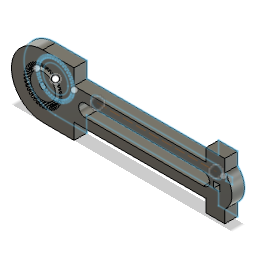
top slider mod v1 (Autodesk Fusion 360 design; units mm, degrees)
Autodesk Fusion 360 part; units mm, degrees
sketch "Sketch1" plane through (0, 0, 0) normal (0, 0, 1) x (1, 0, 0)
  line L0 (100.0107, 100.3168) -> (205.0107, 100.3168)
  line L1 (205.0107, 75.3168) -> (100.0107, 75.3168)
  line L2 (100.0107, 100.3168) -> (100.0107, 112.8168)
  line L3 (100.0107, 112.8168) -> (75.2033, 112.8168)
  line L4 (75.1963, 62.8169) -> (100.0107, 62.8169)
  line L5 (100.0107, 62.8169) -> (100.0107, 75.3168)
  arc A0 (75.2033, 112.8168) -> (75.1963, 62.8169) centre (75.2032, 87.8168) ccw
  circle A1 centre (75.2032, 87.8168) radius 10
  line L6 (74.5404, 102.8022) -> (74.8532, 100.8268)
  line L7 (74.8532, 100.8268) -> (75.5532, 100.8268)
  line L8 (75.5532, 100.8268) -> (75.9001, 102.8007)
  line L9 (72.1452, 102.5018) -> (72.7708, 100.6022)
  line L10 (72.7708, 100.6022) -> (73.4618, 100.7145)
  line L11 (73.4618, 100.7145) -> (73.4875, 102.7184)
  line L12 (69.8292, 101.8211) -> (70.7514, 100.0464)
  line L13 (70.7514, 100.0464) -> (71.4154, 100.2681)
  line L14 (71.4154, 100.2681) -> (71.1193, 102.2502)
  line L15 (67.6523, 100.7777) -> (68.8473, 99.1739)
  line L16 (68.8473, 99.1739) -> (69.4671, 99.4993)
  line L17 (69.4671, 99.4993) -> (68.8569, 101.4082)
  line L18 (65.671, 99.3986) -> (67.1078, 98.0073)
  line L19 (67.1078, 98.0073) -> (67.6674, 98.4278)
  line L20 (67.6674, 98.4278) -> (66.7589, 100.2142)
  line L21 (63.9366, 97.7196) -> (65.578, 96.5767)
  line L22 (65.578, 96.5767) -> (66.0629, 97.0816)
  line L23 (66.0629, 97.0816) -> (64.8796, 98.6991)
  line L24 (62.494, 95.784) -> (64.2974, 94.9193)
  line L25 (64.2974, 94.9193) -> (64.6951, 95.4954)
  line L26 (64.6951, 95.4954) -> (63.2677, 96.9021)
  line L27 (61.3806, 93.6422) -> (63.2993, 93.0779)
  line L28 (63.2993, 93.0779) -> (63.5994, 93.7103)
  line L29 (63.5994, 93.7103) -> (61.9648, 94.8699)
  line L30 (60.6251, 91.3494) -> (62.6095, 91.1003)
  line L31 (62.6095, 91.1003) -> (62.8043, 91.7726)
  line L32 (62.8043, 91.7726) -> (61.0049, 92.6549)
  line L33 (60.2472, 88.9652) -> (62.2459, 89.0376)
  line L34 (62.2459, 89.0376) -> (62.3303, 89.7325)
  line L35 (62.3303, 89.7325) -> (60.4127, 90.3147)
  line L36 (60.2567, 86.5512) -> (62.2179, 86.9433)
  line L37 (62.2179, 86.9433) -> (62.1897, 87.6427)
  line L38 (62.1897, 87.6427) -> (60.2035, 87.9098)
  line L39 (60.6533, 84.17) -> (62.5262, 84.8716)
  line L40 (62.5262, 84.8716) -> (62.3862, 85.5574)
  line L41 (62.3862, 85.5574) -> (60.3828, 85.5025)
  line L42 (61.4267, 81.8832) -> (63.1628, 82.8762)
  line L43 (63.1628, 82.8762) -> (62.9146, 83.5307)
  line L44 (62.9146, 83.5307) -> (60.946, 83.1551)
  line L45 (62.5569, 79.7502) -> (64.1113, 81.0088)
  line L46 (64.1113, 81.0088) -> (63.7613, 81.615)
  line L47 (63.7613, 81.615) -> (61.8784, 80.9284)
  line L48 (64.0147, 77.826) -> (65.347, 79.3176)
  line L49 (65.347, 79.3176) -> (64.9043, 79.8599)
  line L50 (64.9043, 79.8599) -> (63.156, 78.8802)
  line L51 (65.7622, 76.1606) -> (66.838, 77.8467)
  line L52 (66.838, 77.8467) -> (66.3141, 78.3108)
  line L53 (66.3141, 78.3108) -> (64.7455, 77.0634)
  line L54 (67.7543, 74.7971) -> (68.5457, 76.6339)
  line L55 (68.5457, 76.6339) -> (67.954, 77.008)
  line L56 (67.954, 77.008) -> (66.6059, 75.5251)
  line L57 (69.9392, 73.7708) -> (70.4258, 75.7108)
  line L58 (70.4258, 75.7108) -> (69.7818, 75.9851)
  line L59 (69.7818, 75.9851) -> (68.689, 74.3052)
  line L60 (72.2605, 73.1083) -> (72.4296, 75.1012)
  line L61 (72.4296, 75.1012) -> (71.7499, 75.2687)
  line L62 (71.7499, 75.2687) -> (70.9408, 73.4352)
  line L63 (74.6581, 72.8268) -> (74.5052, 74.8209)
  line L64 (74.5052, 74.8209) -> (73.8075, 74.8772)
  line L65 (73.8075, 74.8772) -> (73.3029, 72.9377)
  line L66 (77.0697, 72.9334) -> (76.599, 74.8772)
  line L67 (76.599, 74.8772) -> (75.9012, 74.8209)
  line L68 (75.9012, 74.8209) -> (75.7143, 72.8256)
  line L69 (79.433, 73.4256) -> (78.6565, 75.2687)
  line L70 (78.6565, 75.2687) -> (77.9769, 75.1012)
  line L71 (77.9769, 75.1012) -> (78.1125, 73.1017)
  line L72 (81.6867, 74.2904) -> (80.6247, 75.9851)
  line L73 (80.6247, 75.9851) -> (79.9807, 75.7108)
  line L74 (79.9807, 75.7108) -> (80.4353, 73.7589)
  line L75 (83.7726, 75.5056) -> (82.4524, 77.008)
  line L76 (82.4524, 77.008) -> (81.8608, 76.6339)
  line L77 (81.8608, 76.6339) -> (82.6226, 74.7802)
  line L78 (85.6365, 77.0397) -> (84.0924, 78.3108)
  line L79 (84.0924, 78.3108) -> (83.5685, 77.8467)
  line L80 (83.5685, 77.8467) -> (84.6177, 76.1392)
  line L81 (87.2301, 78.8528) -> (85.5022, 79.8599)
  line L82 (85.5022, 79.8599) -> (85.0595, 79.3176)
  line L83 (85.0595, 79.3176) -> (86.369, 77.8006)
  line L84 (88.5123, 80.8982) -> (86.6452, 81.615)
  line L85 (86.6452, 81.615) -> (86.2952, 81.0088)
  line L86 (86.2952, 81.0088) -> (87.8312, 79.7215)
  line L87 (89.4498, 83.1227) -> (87.4919, 83.5307)
  line L88 (87.4919, 83.5307) -> (87.2436, 82.8762)
  line L89 (87.2436, 82.8762) -> (88.9662, 81.852)
  line L90 (90.0183, 85.4688) -> (88.0203, 85.5574)
  line L91 (88.0203, 85.5574) -> (87.8803, 84.8716)
  line L92 (87.8803, 84.8716) -> (89.7448, 84.1369)
  line L93 (90.2031, 87.8757) -> (88.2167, 87.6427)
  line L94 (88.2167, 87.6427) -> (88.1885, 86.9433)
  line L95 (88.1885, 86.9433) -> (90.1468, 86.5172)
  line L96 (89.9994, 90.2811) -> (88.0761, 89.7325)
  line L97 (88.0761, 89.7325) -> (88.1605, 89.0376)
  line L98 (88.1605, 89.0376) -> (90.1618, 88.9312)
  line L99 (89.4125, 92.6227) -> (87.6022, 91.7726)
  line L100 (87.6022, 91.7726) -> (87.7969, 91.1003)
  line L101 (87.7969, 91.1003) -> (89.7893, 91.3163)
  line L102 (88.4576, 94.8398) -> (86.807, 93.7103)
  line L103 (86.807, 93.7103) -> (87.1071, 93.0779)
  line L104 (87.1071, 93.0779) -> (89.0391, 93.6107)
  line L105 (87.1594, 96.875) -> (85.7114, 95.4954)
  line L106 (85.7114, 95.4954) -> (86.109, 94.9193)
  line L107 (86.109, 94.9193) -> (87.9305, 95.7551)
  line L108 (85.5516, 98.6756) -> (84.3436, 97.0816)
  line L109 (84.3436, 97.0816) -> (84.8285, 96.5767)
  line L110 (84.8285, 96.5767) -> (86.4923, 97.6939)
  line L111 (83.6757, 100.1949) -> (82.7391, 98.4278)
  line L112 (82.7391, 98.4278) -> (83.2987, 98.0073)
  line L113 (83.2987, 98.0073) -> (84.7617, 99.3769)
  line L114 (81.5804, 101.3937) -> (80.9393, 99.4993)
  line L115 (80.9393, 99.4993) -> (81.5592, 99.1739)
  line L116 (81.5592, 99.1739) -> (82.7836, 100.7605)
  line L117 (79.3199, 102.2409) -> (78.9911, 100.2681)
  line L118 (78.9911, 100.2681) -> (79.6551, 100.0464)
  line L119 (79.6551, 100.0464) -> (80.6091, 101.8089)
  line L120 (76.9528, 102.7145) -> (76.9447, 100.7145)
  line L121 (76.9447, 100.7145) -> (77.6356, 100.6022)
  line L122 (77.6356, 100.6022) -> (78.2946, 102.4948)
  arc A2 (79.3199, 102.2409) -> (78.2946, 102.4948) centre (75.2032, 87.8168) ccw
  arc A3 (81.5804, 101.3937) -> (80.6091, 101.8089) centre (75.2032, 87.8168) ccw
  arc A4 (83.6757, 100.1949) -> (82.7836, 100.7605) centre (75.2032, 87.8168) ccw
  arc A5 (85.5516, 98.6756) -> (84.7617, 99.3769) centre (75.2032, 87.8168) ccw
  arc A6 (87.1594, 96.875) -> (86.4923, 97.6939) centre (75.2032, 87.8168) ccw
  arc A7 (88.4576, 94.8398) -> (87.9305, 95.7551) centre (75.2032, 87.8168) ccw
  arc A8 (89.4125, 92.6227) -> (89.0391, 93.6107) centre (75.2032, 87.8168) ccw
  arc A9 (89.9994, 90.2811) -> (89.7893, 91.3163) centre (75.2032, 87.8168) ccw
  arc A10 (90.1999, 87.5016) -> (90.1618, 88.9312) centre (75.2032, 87.8168) ccw
  arc A11 (90.0183, 85.4688) -> (90.1468, 86.5172) centre (75.2032, 87.8168) ccw
  arc A12 (89.4498, 83.1227) -> (89.7448, 84.1369) centre (75.2032, 87.8168) ccw
  arc A13 (88.5123, 80.8982) -> (88.9662, 81.852) centre (75.2032, 87.8168) ccw
  arc A14 (87.2301, 78.8528) -> (87.8312, 79.7215) centre (75.2032, 87.8168) ccw
  arc A15 (85.6365, 77.0397) -> (86.369, 77.8006) centre (75.2032, 87.8168) ccw
  arc A16 (83.7726, 75.5056) -> (84.6177, 76.1392) centre (75.2032, 87.8168) ccw
  arc A17 (81.6867, 74.2904) -> (82.6226, 74.7802) centre (75.2032, 87.8168) ccw
  arc A18 (79.433, 73.4256) -> (80.4353, 73.7589) centre (75.2032, 87.8168) ccw
  arc A19 (77.0697, 72.9334) -> (78.1125, 73.1017) centre (75.2032, 87.8168) ccw
  arc A20 (74.6581, 72.8268) -> (75.7143, 72.8256) centre (75.2032, 87.8168) ccw
  arc A21 (72.2605, 73.1083) -> (73.3029, 72.9377) centre (75.2032, 87.8168) ccw
  arc A22 (69.9392, 73.7708) -> (70.9408, 73.4352) centre (75.2032, 87.8168) ccw
  arc A23 (67.7543, 74.7971) -> (68.689, 74.3052) centre (75.2032, 87.8168) ccw
  arc A24 (65.7622, 76.1606) -> (66.6059, 75.5251) centre (75.2032, 87.8168) ccw
  arc A25 (64.0147, 77.826) -> (64.7455, 77.0634) centre (75.2032, 87.8168) ccw
  arc A26 (62.5569, 79.7502) -> (63.156, 78.8802) centre (75.2032, 87.8168) ccw
  arc A27 (61.4267, 81.8832) -> (61.8784, 80.9284) centre (75.2032, 87.8168) ccw
  arc A28 (60.6533, 84.17) -> (60.946, 83.1551) centre (75.2032, 87.8168) ccw
  arc A29 (60.2567, 86.5512) -> (60.3828, 85.5025) centre (75.2032, 87.8168) ccw
  arc A30 (60.2472, 88.9652) -> (60.2065, 87.5016) centre (75.2032, 87.8168) ccw
  arc A31 (60.6251, 91.3494) -> (60.4127, 90.3147) centre (75.2032, 87.8168) ccw
  arc A32 (61.3806, 93.6422) -> (61.0049, 92.6549) centre (75.2032, 87.8168) ccw
  arc A33 (62.494, 95.784) -> (61.9648, 94.8699) centre (75.2032, 87.8168) ccw
  arc A34 (63.9366, 97.7196) -> (63.2677, 96.9021) centre (75.2032, 87.8168) ccw
  arc A35 (65.671, 99.3986) -> (64.8796, 98.6991) centre (75.2032, 87.8168) ccw
  arc A36 (67.6523, 100.7777) -> (66.7589, 100.2142) centre (75.2032, 87.8168) ccw
  arc A37 (69.8292, 101.8211) -> (68.8569, 101.4082) centre (75.2032, 87.8168) ccw
  arc A38 (72.1452, 102.5018) -> (71.1193, 102.2502) centre (75.2032, 87.8168) ccw
  arc A39 (76.9528, 102.7145) -> (75.9001, 102.8007) centre (75.2032, 87.8168) ccw
  arc A40 (74.5404, 102.8022) -> (73.4875, 102.7184) centre (75.2032, 87.8168) ccw
  line L123 (211, 90.3168) -> (216, 90.3168)
  line L124 (216, 90.3168) -> (216, 85.3168)
  line L125 (216, 85.3168) -> (211, 85.3168)
  line L126 (211, 85.3168) -> (211, 90.3168)
  arc A41 (220.0107, 75.3168) -> (220.0107, 100.3168) centre (208.894, 87.8168) ccw
  line L127 (220.0107, 100.3168) -> (220.0107, 110.3168)
  line L128 (220.0107, 110.3168) -> (205.0107, 110.3168)
  line L129 (220.0107, 75.3168) -> (220.0107, 65.3168)
  line L130 (220.0107, 65.3168) -> (205.0107, 65.3168)
  line L131 (108.6281, 82.8168) -> (202.9676, 82.8168)
  arc A42 (202.9676, 82.8168) -> (202.9676, 92.8168) centre (202.9676, 87.8168) ccw
  line L132 (202.9676, 92.8168) -> (108.6281, 92.8168)
  arc A43 (108.6281, 92.8168) -> (108.6281, 82.8168) centre (108.6281, 87.8168) ccw
  line L133 (108.6281, 87.8168) -> (202.9676, 87.8168) construction
  line L134 (205.0107, 110.3168) -> (205.0107, 100.3168)
  line L135 (205.0107, 75.3168) -> (205.0107, 65.3168)
  circle A44 centre (75.2032, 87.8168) radius 2.5
  dimension "d1" = 120
  dimension "d4" = 25
  dimension "d8" = 50
  dimension "d9" = 20
  dimension "d10" = 30
  dimension "d11" = 2
  dimension "d12" = 0.7
  dimension "d16" = 360
  dimension "d17" = 5
  dimension "d18" = 5
  dimension "d21" = 15
  dimension "d22" = 10
  dimension "d23" = 10
  dimension "d24" = 10
  dimension "d25" = 5
  constraint horizontal L0
  constraint horizontal L1
  constraint perpendicular L0 L2
  constraint perpendicular L2 L3
  constraint perpendicular L2 L4
  constraint perpendicular L1 L5
  constraint concentric A0 A1
  constraint concentric A1 A39
  constraint coincident L6.start A39
  constraint concentric A2 A39
  constraint concentric A3 A39
  constraint concentric A4 A39
  constraint concentric A5 A39
  constraint concentric A6 A39
  constraint concentric A7 A39
  constraint concentric A8 A39
  constraint concentric A9 A39
  constraint concentric A10 A39
  constraint concentric A11 A39
  constraint concentric A12 A39
  constraint concentric A13 A39
  constraint concentric A14 A39
  constraint concentric A15 A39
  constraint concentric A16 A39
  constraint concentric A17 A39
  constraint concentric A18 A39
  constraint concentric A19 A39
  constraint concentric A20 A39
  constraint concentric A21 A39
  constraint concentric A22 A39
  constraint concentric A23 A39
  constraint concentric A24 A39
  constraint concentric A25 A39
  constraint concentric A26 A39
  constraint concentric A27 A39
  constraint concentric A28 A39
  constraint concentric A29 A39
  constraint concentric A30 A39
  constraint concentric A31 A39
  constraint concentric A32 A39
  constraint concentric A33 A39
  constraint concentric A34 A39
  constraint concentric A35 A39
  constraint concentric A36 A39
  constraint concentric A37 A39
  constraint concentric A38 A39
  constraint concentric A39 A40
  constraint horizontal L123
  constraint vertical L124
  constraint horizontal L125
  constraint vertical L126
  constraint perpendicular L1 L134
  constraint perpendicular L0 L127
  constraint perpendicular L128 L134
  constraint perpendicular L1 L129
  constraint perpendicular L130 L134
  constraint tangent L131 A42
  constraint tangent A42 L132
  constraint parallel L131 L132
  constraint tangent L132 A43
  constraint tangent L131 A43
  constraint concentric A24 A44
  measures "d1" distance of L0.start A41.end
  measures "d4" distance of A41.end A41.start
  measures "d8" diameter of A0
  measures "d9" diameter of A1
  measures "d10" diameter of A39
  measures "d11" distance of L6.start L6.end
  measures "d12" distance of L6.end L7.end
  measures "d17" distance of L123.start L123.end
  measures "d18" distance of L123.end L124.end
  measures "d21" distance of A41.end L134
  measures "d22" distance of A41.end L127.end
  measures "d23" distance of A41.start L129.end
  measures "d24" distance of L131 L132
  measures "d25" diameter of A44
extrude "Extrude1" add sketch "Sketch1" along normal blind 10 makes body 1 at (85.7365, 66.6934, 0) makes body 2 at (85.1908, 87.3184, 6.6667)
extrude "Extrude2" add sketch "Sketch1" along normal blind 2 contours L6 L7 L8 L9 L10 L11 L12 L13 L14 L15 L16 L17 L18 L19 L20 L21 L22 L23 L24 L25 L26 L27 L28 L29 L30 L31 L32 L33 L34 L35 L36 L37 L38 L39 L40 L41 L42 L43 L44 L45 L46 L47 L48 L49 L50 L51 L52 L53 L54 L55 L56 L57 L58 L59 L60 L61 L62 L63 L64 L65 L66 L67 L68 L69 L70 L71 L72 L73 L74 L75 L76 L77 L78 L79 L80 L81 L82 L83 L84 L85 L86 L87 L88 L89 L90 L91 L92 L93 L94 L95 L96 L97 L98 L99 L100 L101 L102 L103 L104 L105 L106 L107 L108 L109 L110 L111 L112 L113 L114 L115 L116 L117 L118 L119 L120 L121 L122 A2 A3 A4 A5 A6 A7 A8 A9 A10 A11 A12 A13 A14 A15 A16 A17 A18 A19 A20 A21 A22 A23 A24 A25 A26 A27 A28 A29 A30 A31 A32 A33 A34 A35 A36 A37 A38 A39 A40 bodies 1 2
